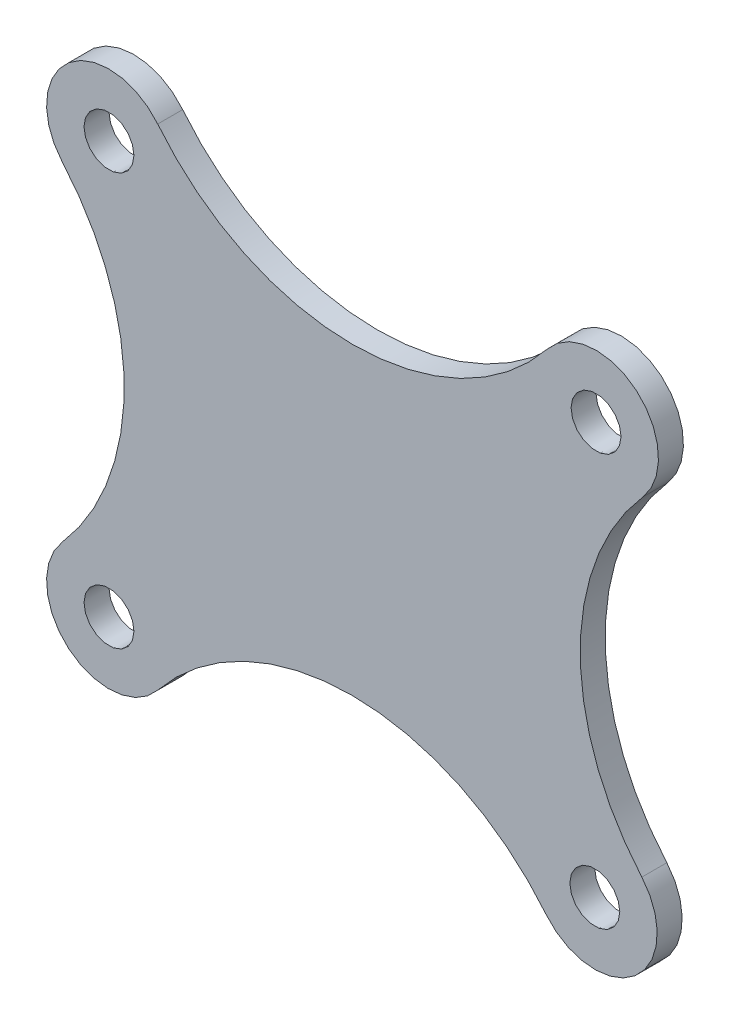
# Autodesk Inventor part: ts_holder
Saved by Autodesk Inventor 2024 (Build 280153000, 153)
## iProperties
Created: 2023-05-15
Part Number: ts_holder
Material: Типовые
Document SubType Name: Modeling
Designer: user
Density: 1 g/cm^3
Appearance: По умолчанию
Author: user
Autodesk Inventor part; units mm, degrees
ref_plane "YZ Plane" through (0, 0, 0) normal (1, 0, 0) x (0, 1, 0)
ref_plane "XZ Plane" through (0, 0, 0) normal (0, 1, 0) x (-1, 0, 0)
ref_plane "XY Plane" through (0, 0, 0) normal (0, 0, 1) x (1, 0, 0)
sketch "Эскиз1" plane through (0, 0, 0) normal (0, 0, 1) x (1, 0, 0)
  circle A0 centre (0, 0) radius 2 projected
  circle A1 centre (-39, 0) radius 2 projected
  arc A2 (-35.1, 3.1289) -> (-42.7563, -3.3) centre (-39, 0) ccw
  arc A3 (-42.7563, -29.7) -> (-35.11, -36.1413) centre (-39, -33) ccw
  arc A4 (3.7463, -3.3114) -> (-3.9, 3.1289) centre (0, 0) ccw
  arc A5 (-3.99, -36.1413) -> (3.6663, -29.7114) centre (-0.1, -33) ccw
  arc A6 (-35.1, 3.1289) -> (-3.9, 3.1289) centre (-19.5, 15.6445) ccw
  arc A7 (3.7463, -3.3114) -> (3.6663, -29.7114) centre (18.7315, -16.5569) ccw
  arc A8 (-42.7563, -29.7) -> (-42.7563, -3.3) centre (-57.7816, -16.5) ccw
  circle A9 centre (-39, -33) radius 2
  circle A10 centre (-0.1, -33) radius 2
  arc A11 (-3.99, -36.1413) -> (-35.11, -36.1413) centre (-19.55, -48.7066) ccw
  point P0 (0, 0)
  dimension "d1" = 5
  dimension "d2" = 20
  constraints: 16 point on circle, 10 centre point, 8 tangent, 6 equal radius, 4 coincident, 4 other
  measures "d1" radius of A3
  measures "d2" radius of A6
extrude "Выдавливание1" add sketch "Эскиз1" along normal blind 2
